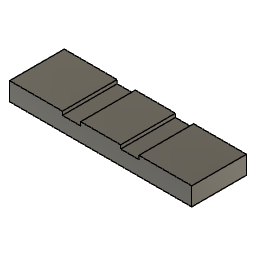
plate with trench v1 (Autodesk Fusion 360 design; units mm, degrees)
Autodesk Fusion 360 part; units mm, degrees
sketch "Sketch1" plane through (0, 0, 0) normal (0, 0, 1) x (1, 0, 0)
  line L0 (0, 0) -> (63.5, 0)
  line L1 (63.5, 0) -> (63.5, 19.05)
  line L2 (63.5, 19.05) -> (0, 19.05)
  line L3 (0, 19.05) -> (0, 0)
  dimension "d1" = 63.5
  dimension "d2" = 19.05
  constraint horizontal L0
  constraint vertical L1
  constraint horizontal L2
  constraint vertical L3
  constraint coincident L0.start L3.end
  measures "d1" distance of L0.start L0.end
  measures "d2" distance of L0.start L2.end
extrude "Extrude1" add sketch "Sketch1" along normal blind 6.35
sketch "Sketch2" plane through (0, 0, 6.35) normal (0, 0, 1) x (-1, 0, 0)
  line L0 (0, -19.05) -> (0, 0)
  line L1 (0, 0) -> (-63.5, 0)
  line L2 (-63.5, 0) -> (-63.5, -19.05)
  line L3 (-63.5, -19.05) -> (0, -19.05)
  line L4 (0, 0) -> (0, -9.525)
  line L5 (0, -19.05) -> (-9.2075, -19.05)
  circle A0 centre (-9.2075, -9.4653) radius 4.0005
  line L6 (0, -19.05) -> (-18.415, -19.05)
  line L7 (-1.154, -19.05) -> (-2.7137, -19.7589)
  line L8 (0, -19.05) -> (-24.765, -19.05)
  line L9 (-24.765, -19.05) -> (-18.415, -19.05)
  line L10 (-18.415, -19.05) -> (-18.415, 0)
  line L11 (-18.415, 0) -> (-24.765, 0)
  line L12 (-24.765, 0) -> (-24.765, -19.05)
  line L13 (-24.765, -19.05) -> (-38.735, -19.05)
  line L14 (-63.5, -19.05) -> (-54.2925, -19.05)
  line L15 (-63.5, -19.05) -> (-45.085, -19.05)
  line L16 (-63.5, 0) -> (-63.5, -9.525)
  circle A1 centre (-54.2925, -9.6525) radius 4.0005
  line L17 (-38.735, -19.05) -> (-38.735, 0)
  line L18 (-45.085, -19.05) -> (-45.085, 0)
  line L19 (-45.085, -19.05) -> (-38.735, -19.05)
  line L20 (-38.735, -19.05) -> (-38.735, 0)
  line L21 (-38.735, 0) -> (-45.085, 0)
  line L22 (-45.085, 0) -> (-45.085, -19.05)
  dimension "d5" = 9.525
  dimension "d6" = 9.2075
  dimension "d7" = 8.001
  dimension "d8" = 18.415
  dimension "d9" = 24.765
  dimension "d10" = 6.35
  dimension "d11" = 19.05
  dimension "d12" = 13.97
  dimension "d13" = 9.2075
  dimension "d14" = 18.415
  dimension "d15" = 9.525
  dimension "d16" = 8.001
  constraint coincident L0.end L1.start
  constraint midpoint L0 L4.end
  constraint coincident L0.start L3.end
  constraint perpendicular L0 L5
  constraint perpendicular L0 L6
  constraint coincident L6 L7.start
  constraint parallel L3 L8
  constraint horizontal L9
  constraint vertical L10
  constraint horizontal L11
  constraint vertical L12
  constraint coincident L3 L13.end
  constraint coincident L2.end L3.start
  constraint perpendicular L2 L14
  constraint perpendicular L2 L15
  constraint coincident L1.end L2.start
  constraint perpendicular L1 L16
  constraint coincident L1 L17.end
  constraint perpendicular L1 L17
  constraint coincident L1 L18.end
  constraint perpendicular L1 L18
  constraint horizontal L19
  constraint vertical L20
  constraint horizontal L21
  constraint vertical L22
  measures "d5" distance of L0.end L4.end
  measures "d6" distance of L0.start L5.end
  measures "d7" diameter of A0
  measures "d8" distance of L0.start L6.end
  measures "d9" distance of L0.start L8.end
  measures "d10" distance of L8.end L6.end
  measures "d11" distance of L8.end L11.end
  measures "d12" distance of L8.end L13.end
  measures "d13" distance of L2.end L14.end
  measures "d14" distance of L2.end L15.end
  measures "d15" distance of L1.end L16.end
  measures "d16" diameter of A1
extrude "Extrude2" cut sketch "Sketch2" against normal blind 1.27 contours L1 L3 L8 L9 L10 L11 L12 | L1 L3 L17 L18 L19 L20 L21 L22
